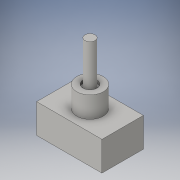
# Autodesk Inventor part: mcdave_switch
Saved by Autodesk Inventor 2016 (Build 200138000, 138)
## iProperties
Created: 2017-09-07
Part Number: mcdave_switch
Material: Generic
Document SubType Name: Modeling
Designer: student
Density: 1 g/cm^3
Appearance: Default
Author: student
Autodesk Inventor part; units mm, degrees
ref_plane "YZ Plane" through (0, 0, 0) normal (1, 0, 0) x (0, 1, 0)
ref_plane "XZ Plane" through (0, 0, 0) normal (0, 1, 0) x (-1, 0, 0)
ref_plane "XY Plane" through (0, 0, 0) normal (0, 0, 1) x (1, 0, 0)
sketch "Sketch1" plane through (0, 0, 0) normal (0, 0, 1) x (1, 0, 0)
  line L0 (-12.0255, 5.2117) -> (16.8797, 5.2117)
  line L1 (16.8797, 5.2117) -> (16.8797, -7.7423)
  line L2 (16.8797, -7.7423) -> (-12.0255, -7.7423)
  line L3 (-12.0255, -7.7423) -> (-12.0255, 5.2117)
  point P0 (0, 0)
  dimension "d0" = 12.954
  dimension "d1" = 28.9052
  constraints: 8 end point, 2 parallel, 1 horizontal, 1 perpendicular
  measures "d0" distance of L0.end L1.end
  measures "d1" distance of L1.end L2.end
extrude "Extrusion1" add sketch "Sketch1" along normal blind 18.3388
sketch "Sketch2" plane through (-12.0255, 5.2117, 0) normal (0, 1, 0) x (1, 0, 0)
  line L0 (0, 0) -> (28.9052, 0) projected
  line L1 (28.9052, -18.3388) -> (0, -18.3388) projected
  line L2 (0, 0) -> (0, -18.3388) projected
  circle A0 centre (14.4526, -9.1694) radius 5.8547
  point P0 (12.0255, 0)
  dimension "d4" = 11.7094
  constraints: 1 centre point
  measures "d4" diameter of A0
extrude "Extrusion2" add sketch "Sketch2" along normal blind 9.3472
sketch "Sketch3" plane through (2.4271, 14.5589, 9.1694) normal (0, 1, 0) x (1, 0, 0)
  circle A0 centre (0, 0) radius 3.0988
  point P0 (-2.4271, 9.1694)
  dimension "d7" = 6.1976
  constraints: 1 centre point
  measures "d7" diameter of A0
extrude "Extrusion3" cut sketch "Sketch3" against normal blind 1.27
sketch "Sketch4" plane through (2.4271, 13.2889, 9.1694) normal (0, 1, 0) x (1, 0, 0)
  circle A0 centre (0, 0) radius 2.2352
  point P0 (-2.4271, 9.1694)
  dimension "d10" = 4.4704
  constraints: 1 centre point
  measures "d10" diameter of A0
extrude "Extrusion4" add sketch "Sketch4" along normal blind 19.0754
body "Solid1"
